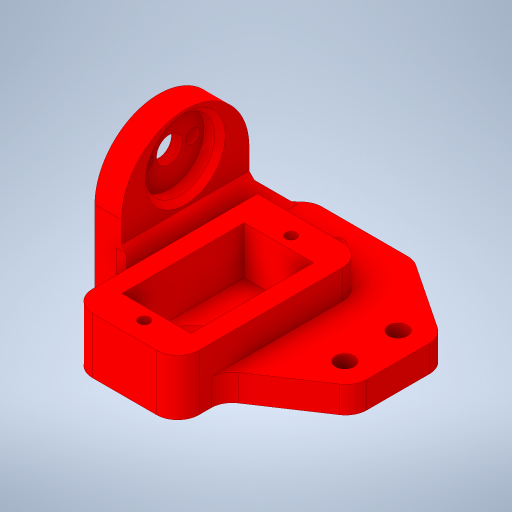
# Autodesk Inventor part: grip_base
Saved by Autodesk Inventor 2023 (Build 270158000, 158)
## iProperties
Part Number: grip_base
Material: PLA plastic
Document SubType Name: Modeling
Designer: denyh
Density: 1.25 g/cm^3
Appearance: Generic
Mass: 16.9819 g
Surface Area: 78.9348 cm^2
Volume: 16.0207 cm^3
Author: denyh
Autodesk Inventor part; units mm, degrees
ref_plane "YZ Plane" through (0, 0, 0) normal (1, 0, 0) x (0, 1, 0)
ref_plane "XZ Plane" through (0, 0, 0) normal (0, 1, 0) x (-1, 0, 0)
ref_plane "XY Plane" through (0, 0, 0) normal (0, 0, 1) x (1, 0, 0)
sketch "Náčrt1" plane through (0, 0, 0) normal (0, 0, 1) x (1, 0, 0)
  line L0 (0, 0) -> (18.8, 0)
  line L1 (18.8, 0) -> (33.8102, -10.0068)
  line L2 (33.8102, -10.0068) -> (33.8102, -26.0068)
  line L3 (33.8102, -26.0068) -> (18.8, -36.0135)
  line L4 (18.8, -36.0135) -> (18.8, -44.4135)
  line L5 (18.8, -44.4135) -> (-1.2, -44.4135)
  line L6 (-1.2, -44.4135) -> (-1.2, -36.0135)
  line L7 (-1.2, -36.0135) -> (-11.1999, -26.0136)
  line L8 (-11.1999, -26.0136) -> (-11.1999, -6.0136)
  line L9 (-11.1999, -6.0136) -> (-6.696, -6.0136)
  line L10 (-6.696, -6.0136) -> (0, 0)
  line L11 (0, 0) -> (8.815, 0)
  line L12 (8.815, 0) -> (8.815, -5)
  circle A0 centre (8.815, -5) radius 1.75
  line L13 (33.8102, -10.0068) -> (33.8102, -13.0068)
  line L14 (33.8102, -13.0068) -> (28.8102, -13.0068)
  circle A1 centre (28.8102, -13.0068) radius 1.75
  line L15 (33.8102, -18.0068) -> (26.6273, -18.0068)
  circle A2 centre (28.8102, -23.0068) radius 1.75
  line L16 (8.8, -44.4135) -> (8.8, -31.9135)
  circle A3 centre (8.8, -31.9135) radius 5.4
  dimension "d0" = 18.8
  dimension "d1" = 18.04
  dimension "d2" = 146.31
  dimension "d3" = 16
  dimension "d4" = 18.04
  dimension "d5" = 123.69
  dimension "d6" = 8.4
  dimension "d7" = 20
  dimension "d8" = 14.142
  dimension "d9" = 135
  dimension "d10" = 20
  dimension "d12" = 9
  dimension "d13" = 8.815
  dimension "d14" = 5
  dimension "d15" = 3.5
  dimension "d16" = 3
  dimension "d17" = 5
  dimension "d18" = 3.5
  dimension "d19" = 12.5
  dimension "d20" = 10.8
  constraints: 34 end point, 5 vertical, 4 centre point, 4 horizontal, 3 coincident, 2 midpoint, 2 perpendicular, 2 point on line, 1 symmetric about line, 1 other
  measures "d0" distance of L0.start L0.end
  measures "d1" distance of L0.end L1.end
  measures "d2" angle of L0 L1
  measures "d3" distance of L1.end L2.end
  measures "d4" distance of L2.end L3.end
  measures "d5" angle of L2 L3
  measures "d6" distance of L3.end L4.end
  measures "d7" distance of L4.end L5.end
  measures "d8" distance of L6.end L7.end
  measures "d9" angle of L6 L7
  measures "d10" distance of L7.end L8.end
  measures "d12" distance of L9.end L0.start
  measures "d13" distance of L0.start L11.end
  measures "d14" distance of L11.end L12.end
  measures "d15" diameter of A0
  measures "d16" distance of L1.end L13.end
  measures "d17" distance of L13.end L14.end
  measures "d18" diameter of A1
  measures "d19" distance of L16.start L16.end
  measures "d20" diameter of A3
extrude "Vysunutí1" add sketch "Náčrt1" along normal blind 5
sketch "Náčrt2" plane through (0, 0, 5) normal (0, 0, 1) x (1, 0, 0)
  line L0 (18.8, 0) -> (0, 0) projected
  line L1 (18.8, 0) -> (18.8, -9.4)
  line L2 (18.8, -9.4) -> (-1.2, -9.4)
  line L3 (18.8, -44.4135) -> (18.8, -36.0135) projected
  line L4 (18.8, -9.4) -> (18.8, -44.4135)
  line L5 (-1.2, -44.4135) -> (18.8, -44.4135) projected
  line L6 (18.8, -44.4135) -> (-1.2, -44.4135)
  line L7 (-1.2, -36.0135) -> (-1.2, -44.4135) projected
  line L8 (-1.2, -9.4) -> (-1.2, -44.4135)
  dimension "d24" = 9.4
  dimension "d25" = 20
  constraints: 10 end point, 2 collinear, 1 perpendicular, 1 vertical
  measures "d24" distance of L0.start L1.end
  measures "d25" distance of L1.end L2.end
extrude "Vysunutí2" add sketch "Náčrt2" along normal blind 5.5
sketch "Náčrt4" plane through (0, 0, 10.5) normal (0, 0, 1) x (1, 0, 0)
  circle A0 centre (8.8, -31.9135) radius 5.4 projected
  line L0 (8.8, -31.9135) -> (2.3, -31.9135)
  line L1 (8.8, -31.9135) -> (8.8, -38.4135)
  line L2 (8.8, -31.9135) -> (15.3, -31.9135)
  line L3 (15.3, -31.9135) -> (15.3, -38.4135)
  line L4 (15.3, -38.4135) -> (2.3, -38.4135)
  line L5 (2.3, -38.4135) -> (2.3, -31.9135)
  line L6 (2.3, -38.4135) -> (2.3, -15.4135)
  line L7 (2.3, -15.4135) -> (15.3, -15.4135)
  line L8 (15.3, -15.4135) -> (15.3, -31.9135)
  point P0 (0, 0)
  dimension "d42" = 6.5
  dimension "d43" = 6.5
  dimension "d44" = 6.5
  dimension "d45" = 23
  constraints: 18 end point, 4 perpendicular, 2 vertical, 1 collinear, 1 horizontal, 1 point on line
  measures "d42" distance of L0.start L0.end
  measures "d43" distance of L0.start L1.end
  measures "d44" distance of L0.start L2.end
  measures "d45" distance of L4.end L6.end
extrude "Vysunutí4" cut sketch "Náčrt4" against normal blind 9
sketch "Náčrt5" plane through (0, 0, 10.5) normal (0, 0, 1) x (1, 0, 0)
  circle A0 centre (8.8, -31.9135) radius 5.4 projected
  line L0 (8.8, -31.9135) -> (8.8, -40.7135)
  circle A1 centre (8.8, -40.7135) radius 1
  line L1 (15.3, -15.4135) -> (15.3, -38.4135) projected
  line L2 (15.3, -26.9135) -> (6.7604, -26.9135)
  circle A2 centre (8.8, -13.1135) radius 1
  point P0 (0, 0)
  dimension "d48" = 8.8
  dimension "d49" = 2
  constraints: 4 end point, 2 centre point, 1 coincident, 1 midpoint, 1 perpendicular, 1 symmetric about line, 1 vertical, 3 other
  measures "d48" distance of L0.start L0.end
  measures "d49" diameter of A1
extrude "Vysunutí5" cut sketch "Náčrt5" against normal blind 7 contours A1 | A2
fillet "Zaoblení2" radius 4 10 edges at (-11.1999, -26.0136, 2.5) (-1.2, -36.0135, 2.5) (-1.2, -44.4135, 5.25) (18.8, -44.4135, 5.25) (18.8, -9.4, 7.75) (0, 0, 2.5) (18.8, 0, 2.5) (33.8102, -10.0068, 2.5) (33.8102, -26.0068, 2.5) (18.8, -36.0135, 2.5)
fillet "Zaoblení4" radius 4 1 edges at (-6.696, -6.0136, 2.5)
sketch "Sketch6" plane through (0, 0, 5) normal (0, 0, 1) x (1, 0, 0)
  line L0 (33.8102, -23.866) -> (33.8102, -12.1475) projected
  line L1 (33.8102, -18.0068) -> (-11.1999, -18.0068)
  line L2 (-11.1999, -6.0136) -> (-11.1999, -24.3568) projected
  line L3 (-11.1999, -18.0068) -> (-11.1999, -6.0068)
  line L4 (-11.1999, -6.0068) -> (-6.1999, -6.0068)
  line L5 (-6.1999, -6.0068) -> (-6.1999, -30.0068)
  line L6 (-6.1999, -30.0068) -> (-11.1999, -30.0068)
  line L7 (-11.1999, -30.0068) -> (-11.1999, -18.0068)
  point P0 (0, 0)
  dimension "d56" = 12
  dimension "d57" = 5
  dimension "d58" = 24
  constraints: 12 end point, 3 perpendicular, 3 point on line, 1 collinear, 1 horizontal, 1 midpoint
  measures "d56" distance of L1.end L3.end
  measures "d57" distance of L3.end L4.end
  measures "d58" distance of L4.end L5.end
extrude "Extrusion6" add sketch "Sketch6" along normal blind 21
sketch "Sketch7" plane through (0, 0, 5) normal (0, 0, -1) x (-1, 0, 0)
  line L0 (7.9942, -6.0068) -> (11.1999, -6.0068) projected
  line L1 (8.2285, -6.0136) -> (11.1999, -6.0136) projected
  line L2 (11.1999, -6.0068) -> (11.1999, -6.0136) projected
  arc A0 (10.0283, -27.1852) -> (11.1999, -24.3568) centre (7.1999, -24.3568) ccw projected
  line L3 (10.0283, -27.1852) -> (7.2068, -30.0068) projected
  line L4 (11.1999, -30.0068) -> (7.2068, -30.0068) projected
  line L5 (11.1999, -24.3568) -> (11.1999, -30.0068) projected
  arc A1 (5.5558, -4.9896) -> (8.2285, -6.0136) centre (8.2285, -2.0136) ccw projected
  line L6 (8.2285, -6.0136) -> (11.1999, -6.0136) projected
  line L7 (11.1999, -6.0068) -> (11.1999, -6.0136) projected
  line L8 (7.9942, -6.0068) -> (11.1999, -6.0068) projected
  arc A2 (7.9942, -6.0068) -> (8.2285, -6.0136) centre (8.2285, -2.0136) ccw projected
  point P0 (0, 0)
extrude "Extrusion7" add sketch "Sketch7" along normal blind 5
sketch "Sketch8" plane through (-11.1999, -30.0068, 26) normal (-1, 0, 0) x (0, 0, 1)
  line L0 (-26, 0) -> (-26, 24) projected
  line L1 (-26, 12) -> (-8, 12)
  circle A0 centre (-8, 12) radius 2.4
  line L2 (-8, 12) -> (-8, 16.4)
  circle A1 centre (-8, 16.4) radius 1.3
  line L3 (-8, 12) -> (-8, 7.6)
  circle A2 centre (-8, 7.6) radius 1.3
  point P0 (-26, 30.0068)
  dimension "d63" = 18
  dimension "d64" = 4.8
  dimension "d65" = 4.4
  dimension "d66" = 2.6
  dimension "d67" = 4.4
  dimension "d68" = 2.6
  constraints: 6 end point, 3 centre point, 3 coincident, 2 vertical, 1 horizontal, 1 midpoint
  measures "d63" distance of L1.start L1.end
  measures "d64" diameter of A0
  measures "d65" distance of L2.start L2.end
  measures "d66" diameter of A1
  measures "d67" distance of L2.start L3.end
  measures "d68" diameter of A2
fillet "Fillet6" radius 12 2 edges at (-8.6999, -30.0068, 26) (-8.6999, -6.0068, 26)
extrude "Extrusion8" cut sketch "Sketch8" against normal blind 10
sketch "Sketch9" plane through (-6.1999, -30.0068, 5) normal (1, 0, 0) x (0, 0, -1)
  circle A0 centre (-13, 12) radius 2.4 projected
  circle A1 centre (-13, 12) radius 6.5
  point P0 (5, 30.0068)
  dimension "d72" = 13
  constraints: 1 centre point, 1 coincident
  measures "d72" diameter of A1
extrude "Extrusion9" cut sketch "Sketch9" against normal blind 3
chamfer "Chamfer1" distance 1 angle 45 1 edges at (-6.1999, -18.0068, 24.5)
chamfer "Chamfer2" distance 5 angle 45 1 edges at (-6.1999, -18.0068, 5)
chamfer "Chamfer3" distance 4 angle 45 4 edges at (-3.7, -30.0068, 5) (-6.7033, -30.0068, 5) (-3.7, -6.0068, 5) (-7.097, -6.0068, 5)
